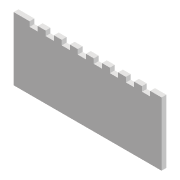
# Autodesk Inventor part: 00_Baseplate_Simmo_side5_v2
Saved by Autodesk Inventor 2022 (Build 260153000, 153)
## iProperties
Created: 2022-08-09
Part Number: 00_Baseplate_Simmo_side5_v2
Material: Generic
Document SubType Name: Modeling
Designer: wanghaoran
Density: 1 g/cm^3
Appearance: Default
Author: wanghaoran
Autodesk Inventor part; units mm, degrees
ref_plane "YZ Plane" through (0, 0, 0) normal (1, 0, 0) x (0, 1, 0)
ref_plane "XZ Plane" through (0, 0, 0) normal (0, 1, 0) x (-1, 0, 0)
ref_plane "XY Plane" through (0, 0, 0) normal (0, 0, 1) x (1, 0, 0)
sketch "Sketch1" plane through (0, 0, 0) normal (0, 0, 1) x (1, 0, 0)
  line L0 (174.3024, 0) -> (174.3024, 6) projected
  line L1 (-10, 0) -> (-10, 6) projected
  line L2 (174.3024, 6) -> (-10, 6)
  line L3 (-10, 6) -> (-10, -73)
  line L4 (-10, -73) -> (174.3024, -73)
  line L5 (174.3024, -73) -> (174.3024, 6)
  point P0 (0, 0)
  dimension "d0" = 79
  constraints: 8 end point, 2 parallel, 1 horizontal, 1 perpendicular
  measures "d0" distance of L3.end L2.end
extrude "Extrusion1" add sketch "Sketch1" along normal blind 6
sketch "Sketch2" plane through (0, 0, 6) normal (0, 0, 1) x (1, 0, 0)
  line L0 (174.3024, 6) -> (-10, 6) projected
  line L1 (150, 0) -> (150, 6) projected
  line L2 (140, 6) -> (140, 0) projected
  line L3 (150.1, 6) -> (139.9, 6)
  line L4 (139.9, 6) -> (139.9, 0)
  line L5 (139.9, 0) -> (150.1, 0)
  line L6 (150.1, 0) -> (150.1, 6)
  point P0 (0, 0)
  dimension "d10" = 10.2
  dimension "d11" = 6
  constraints: 8 end point, 2 parallel, 1 horizontal, 1 perpendicular
  measures "d10" distance of L5.end L4.end
  measures "d11" distance of L4.end L3.end
extrude "Extrusion2" cut sketch "Sketch2" against normal blind 6
pattern_linear "Rectangular Pattern2" count 8 spacing 20 along (-1, 0, 0) of "Extrusion2"
sketch "Sketch3" plane through (0, 0, 6) normal (0, 0, 1) x (1, 0, 0)
  line L0 (160, 0) -> (174.3024, 0) projected
  line L1 (160, 6) -> (160, 0) projected
  line L2 (160, 0) -> (159.9, 0)
  line L3 (159.9, 0) -> (159.9, 6)
  line L4 (159.9, 6) -> (160, 6)
  line L5 (160, 6) -> (160, 0)
  line L6 (174.3024, -73) -> (174.3024, 6) projected
  line L7 (174.3024, 6) -> (150.1, 6) projected
  point P0 (0, 0)
  dimension "d15" = 0.1
  dimension "d16" = 6
  constraints: 8 end point, 2 parallel, 1 horizontal, 1 perpendicular
  measures "d15" distance of L3.end L4.end
  measures "d16" distance of L2.end L3.end
extrude "Extrusion3" cut sketch "Sketch3" against normal blind 6
body "Solid1"
